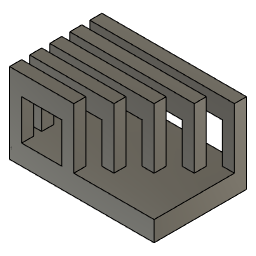
Bridgin test 3 (Autodesk Fusion 360 design; units mm, degrees)
Autodesk Fusion 360 part; units mm, degrees
sketch "Sketch1" plane through (0, 0, 0) normal (0, 0, 1) x (1, 0, 0)
  line L0 (0, 0) -> (36, 0)
  line L1 (36, 0) -> (36, 23)
  line L2 (36, 23) -> (0, 23)
  line L3 (0, 23) -> (0, 0)
  dimension "d1" = 36
  dimension "d2" = 23
  constraint horizontal L0
  constraint vertical L1
  constraint horizontal L2
  constraint vertical L3
  constraint coincident L0.start L3.end
  measures "d1" distance of L0.start L0.end
  measures "d2" distance of L0.start L2.end
extrude "Extrude1" add sketch "Sketch1" along normal blind 5
sketch "Sketch2" plane through (0, 0, 0) normal (0, -1, 0) x (1, 0, 0)
  line L0 (0, 0) -> (36, 0)
  line L1 (36, 0) -> (36, 5)
  line L2 (36, 5) -> (0, 5)
  line L3 (0, 5) -> (0, 0)
  line L4 (0, 5) -> (0, 20)
  line L5 (0, 20) -> (16, 20)
  line L6 (16, 20) -> (16, 5)
  line L7 (16, 5) -> (13, 5)
  line L8 (13, 5) -> (13, 15)
  line L9 (13, 15) -> (3, 15)
  line L10 (3, 15) -> (3, 5)
  dimension "d5" = 15
  dimension "d6" = 3
  dimension "d7" = 10
  dimension "d8" = 10
  constraint coincident L2.end L3.start
  constraint perpendicular L2 L4
  constraint perpendicular L3 L5
  constraint coincident L2 L6.end
  constraint perpendicular L2 L6
  constraint perpendicular L6 L7
  constraint perpendicular L7 L8
  constraint perpendicular L6 L9
  constraint coincident L2 L10.end
  constraint perpendicular L2 L10
  measures "d5" distance of L2.end L4.end
  measures "d6" distance of L6.end L7.end
  measures "d7" distance of L7.end L8.end
  measures "d8" distance of L8.end L9.end
extrude "Extrude2" add sketch "Sketch2" against normal blind 3 contours L2 L4 L5 L6 L7 L8 L9 L10
ref_plane "WorkPlane1" through (18, 5, 10) normal (0, -1, 0) x (1, 0, 0)
sketch "Sketch3" plane through (17.5, 5, 10) normal (0, -1, 0) x (1, 0, 0)
  line L0 (-17.5, -5) -> (-17.5, 10)
  line L1 (-17.5, 10) -> (3.5, 10)
  line L2 (3.5, 10) -> (3.5, -5)
  line L3 (3.5, -5) -> (0.5, -5)
  line L4 (0.5, -5) -> (0.5, 5)
  line L5 (0.5, 5) -> (-14.5, 5)
  line L6 (-14.5, 5) -> (-14.5, -5)
  line L7 (-14.5, -5) -> (-17.5, -5)
  dimension "d12" = 15
  dimension "d13" = 21
  dimension "d14" = 15
  dimension "d15" = 3
  dimension "d16" = 10
  dimension "d17" = 15
  constraint vertical L0
  constraint perpendicular L0 L1
  constraint perpendicular L1 L2
  constraint perpendicular L2 L3
  constraint perpendicular L3 L4
  constraint perpendicular L4 L5
  constraint perpendicular L5 L6
  constraint perpendicular L0 L7
  measures "d12" distance of L0.start L0.end
  measures "d13" distance of L0.end L1.end
  measures "d14" distance of L1.end L2.end
  measures "d15" distance of L2.end L3.end
  measures "d16" distance of L3.end L4.end
  measures "d17" distance of L4.end L5.end
extrude "Extrude3" add sketch "Sketch3" against normal blind 3
ref_plane "WorkPlane2" through (18, 10, 10) normal (0, -1, 0) x (1, 0, 0)
sketch "Sketch4" plane through (18, 10, 10) normal (0, -1, 0) x (1, 0, 0)
  line L0 (-18, -5) -> (-18, 10)
  line L1 (-18, 10) -> (8, 10)
  line L2 (8, 10) -> (8, -5)
  line L3 (8, -5) -> (5, -5)
  line L4 (5, -5) -> (5, 5)
  line L5 (5, 5) -> (-15, 5)
  line L6 (-15, 5) -> (-15, -5)
  line L7 (-15, -5) -> (-18, -5)
  dimension "d21" = 26
  dimension "d22" = 15
  dimension "d23" = 3
  dimension "d24" = 10
  dimension "d25" = 20
  constraint vertical L0
  constraint perpendicular L0 L1
  constraint perpendicular L1 L2
  constraint perpendicular L2 L3
  constraint perpendicular L1 L4
  constraint perpendicular L4 L5
  constraint perpendicular L5 L6
  measures "d21" distance of L0.end L1.end
  measures "d22" distance of L1.end L2.end
  measures "d23" distance of L2.end L3.end
  measures "d24" distance of L3.end L4.end
  measures "d25" distance of L4.end L5.end
extrude "Extrude4" add sketch "Sketch4" against normal blind 3
ref_plane "WorkPlane3" through (18, 15, 10) normal (0, -1, 0) x (1, 0, 0)
sketch "Sketch5" plane through (18, 15, 10) normal (0, -1, 0) x (1, 0, 0)
  line L0 (-18, -5) -> (-18, 10)
  line L1 (-18, 10) -> (13, 10)
  line L2 (13, 10) -> (13, -5)
  line L3 (13, -5) -> (10, -5)
  line L4 (10, -5) -> (10, 5)
  line L5 (10, 5) -> (-15, 5)
  line L6 (-15, 5) -> (-15, -5)
  line L7 (-15, -5) -> (-18, -5)
  dimension "d29" = 31
  dimension "d30" = 15
  dimension "d31" = 3
  dimension "d32" = 10
  dimension "d34" = 25
  constraint vertical L0
  constraint perpendicular L0 L1
  constraint perpendicular L1 L2
  constraint perpendicular L2 L3
  constraint perpendicular L3 L4
  constraint perpendicular L4 L5
  constraint perpendicular L5 L6
  constraint perpendicular L0 L7
  measures "d29" distance of L0.end L1.end
  measures "d30" distance of L1.end L2.end
  measures "d31" distance of L2.end L3.end
  measures "d32" distance of L3.end L4.end
  measures "d34" distance of L4.end L5.end
extrude "Extrude5" add sketch "Sketch5" against normal blind 3
ref_plane "WorkPlane4" through (18, 20, 10) normal (0, -1, 0) x (1, 0, 0)
sketch "Sketch6" plane through (18, 20, 10) normal (0, -1, 0) x (1, 0, 0)
  line L0 (-18, -5) -> (-18, 10)
  line L1 (-18, 10) -> (18, 10)
  line L2 (18, 10) -> (18, -5)
  line L3 (18, -5) -> (15, -5)
  line L4 (15, -5) -> (15, 5)
  line L5 (15, 5) -> (-15, 5)
  line L6 (-15, 5) -> (-15, -5)
  line L7 (-15, -5) -> (-18, -5)
  dimension "d38" = 36
  dimension "d39" = 3
  dimension "d40" = 10
  dimension "d41" = 30
  constraint vertical L0
  constraint perpendicular L0 L1
  constraint perpendicular L1 L2
  constraint perpendicular L2 L3
  constraint perpendicular L3 L4
  constraint perpendicular L4 L5
  constraint perpendicular L5 L6
  constraint perpendicular L0 L7
  measures "d38" distance of L0.end L1.end
  measures "d39" distance of L2.end L3.end
  measures "d40" distance of L3.end L4.end
  measures "d41" distance of L4.end L5.end
extrude "Extrude6" add sketch "Sketch6" against normal blind 3
sketch "Sketch7" plane through (0, 0, 0) normal (-1, 0, 0) x (0, -1, 0)
  line L0 (-23, 0) -> (0, 0)
  line L1 (0, 0) -> (0, 20)
  line L2 (0, 20) -> (-3, 20)
  line L3 (-3, 20) -> (-3, 5)
  line L4 (-3, 5) -> (-5, 5)
  line L5 (-5, 5) -> (-5, 20)
  line L6 (-5, 20) -> (-8, 20)
  line L7 (-8, 20) -> (-8, 5)
  line L8 (-8, 5) -> (-10, 5)
  line L9 (-10, 5) -> (-10, 20)
  line L10 (-10, 20) -> (-13, 20)
  line L11 (-13, 20) -> (-13, 5)
  line L12 (-13, 5) -> (-15, 5)
  line L13 (-15, 5) -> (-15, 20)
  line L14 (-15, 20) -> (-18, 20)
  line L15 (-18, 20) -> (-18, 5)
  line L16 (-18, 5) -> (-20, 5)
  line L17 (-20, 5) -> (-20, 20)
  line L18 (-20, 20) -> (-23, 20)
  line L19 (-23, 20) -> (-23, 0)
  line L20 (-3.0382, 1.4911) -> (-0.1715, 1.4911) construction
  line L21 (-0.1715, 1.4911) -> (-0.1715, 4.4911) construction
  line L22 (-0.1715, 4.4911) -> (-3.0382, 4.4911) construction
  line L23 (-3.0382, 4.4911) -> (-3.0382, 1.4911) construction
  line L24 (-7.9084, 1.3825) -> (-5.0182, 1.3825) construction
  line L25 (-5.0182, 1.3825) -> (-5.0182, 4.3825) construction
  line L26 (-5.0182, 4.3825) -> (-7.9084, 4.3825) construction
  line L27 (-7.9084, 4.3825) -> (-7.9084, 1.3825) construction
  line L28 (-13, 1.5) -> (-9.8945, 1.5) construction
  line L29 (-9.8945, 1.5) -> (-9.8945, 4.5) construction
  line L30 (-9.8945, 4.5) -> (-13, 4.5) construction
  line L31 (-13, 4.5) -> (-13, 1.5) construction
  line L32 (-18.1376, 1.6433) -> (-15.0087, 1.6433) construction
  line L33 (-15.0087, 1.6433) -> (-15.0087, 4.6433) construction
  line L34 (-15.0087, 4.6433) -> (-18.1376, 4.6433) construction
  line L35 (-18.1376, 4.6433) -> (-18.1376, 1.6433) construction
  line L36 (-23, 1.8124) -> (-19.9326, 1.8124) construction
  line L37 (-19.9326, 1.8124) -> (-19.9326, 4.8124) construction
  line L38 (-19.9326, 4.8124) -> (-23, 4.8124) construction
  line L39 (-23, 4.8124) -> (-23, 1.8124) construction
  text T0 "10" font "Arial" height 3 align ink ink in box 0 x 0 at (-3.0382, 1.4911) x (1, 0) y (0, 1) spacing 1 height is em
  text T1 "15" font "Arial" height 3 align ink ink in box 0 x 0 at (-7.9084, 1.3825) x (1, 0) y (0, 1) spacing 1 height is em
  text T2 "20" font "Arial" height 3 align ink ink in box 0 x 0 at (-13, 1.5) x (1, 0) y (0, 1) spacing 1 height is em
  text T3 "25" font "Arial" height 3 align ink ink in box 0 x 0 at (-18.1376, 1.6433) x (1, 0) y (0, 1) spacing 1 height is em
  text T4 "30" font "Arial" height 3 align ink ink in box 0 x 0 at (-23, 1.8124) x (1, 0) y (0, 1) spacing 1 height is em
  constraint perpendicular L20 L21
  constraint parallel L20 L22
  constraint parallel L21 L23
  constraint perpendicular L24 L25
  constraint parallel L24 L26
  constraint parallel L25 L27
  constraint perpendicular L28 L29
  constraint parallel L28 L30
  constraint parallel L29 L31
  constraint perpendicular L32 L33
  constraint parallel L32 L34
  constraint parallel L33 L35
  constraint perpendicular L36 L37
  constraint parallel L36 L38
  constraint parallel L37 L39
  constraint coincident L19 L36.start
extrude "Extrude7" cut sketch "Sketch7" against normal blind 0.5 text T0 T2 T1 T3 T4
